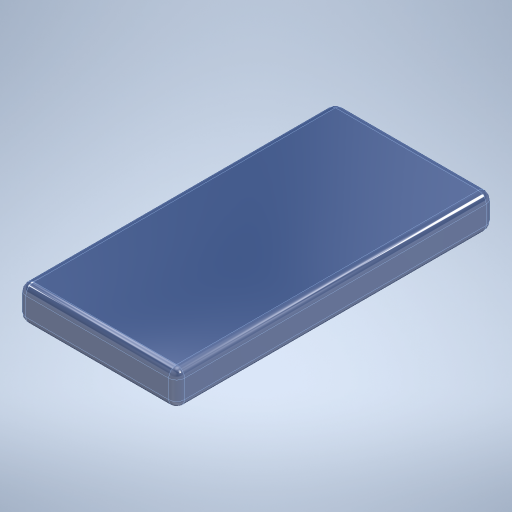
# Autodesk Inventor part: Battery
Saved by Autodesk Inventor 2023 (Build 270158000, 158)
## iProperties
Created: 2023-10-22
Part Number: Battery
Material: Generic
Document SubType Name: Modeling
Designer: Admins
Density: 1 g/cm^3
Appearance: Flaked Satin - Blue
Author: Admins
Autodesk Inventor part; units mm, degrees
ref_plane "YZ Plane" through (0, 0, 0) normal (1, 0, 0) x (0, 1, 0)
ref_plane "XZ Plane" through (0, 0, 0) normal (0, 1, 0) x (-1, 0, 0)
ref_plane "XY Plane" through (0, 0, 0) normal (0, 0, 1) x (1, 0, 0)
sketch "Sketch1" plane through (0, 0, 0) normal (0, 1, 0) x (-1, 0, 0)
  line L0 (-30, 60) -> (30, 60)
  line L1 (30, 60) -> (30, -60)
  line L2 (30, -60) -> (-30, -60)
  line L3 (-30, -60) -> (-30, 60)
  line L4 (-30, 60) -> (30, -60) construction
  line L5 (30, 60) -> (-30, -60) construction
  point P0 (0, 0)
  dimension "d0" = 60
  dimension "d1" = 120
  constraints: 12 end point, 2 midpoint, 2 parallel, 1 horizontal, 1 perpendicular
  measures "d0" distance of L1.end L2.end
  measures "d1" distance of L0.end L1.end
extrude "Extrusion1" add sketch "Sketch1" along normal blind 13
fillet "Fillet1" radius 3 12 edges at (30, 13, 0) (0, 13, 60) (0, 0, 60) (30, 0, 0) (0, 13, -60) (-30, 6.5, -60) (30, 6.5, -60) (30, 6.5, 60) (-30, 6.5, 60) (-30, 13, 0) (-30, 0, 0) (0, 0, -60)
body "Solid1"
